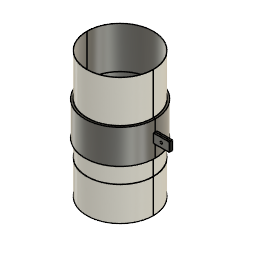
The Avionic Bay (Autodesk Fusion 360 design; units mm, degrees)
part number: 2026-03-09-17-46-28-485
Autodesk Fusion 360 part; units mm, degrees
sketch "Sketch1" plane through (0, 0, 0) normal (0, 0, 1) x (1, 0, 0)
  circle A0 centre (0, 0) radius 29.3705
  dimension "d1" = 58.741
  constraint coincident A0.centre origin
  measures "d1" diameter of A0
extrude "Extrude1" add sketch "Sketch1" along normal blind 112.014 makes body 1
shell "Shell1" thickness 0.1 removed faces 1 at (-8.7113, 2.7886, 112.014) on bodies 1
hole "Hole1" at (0, 0, 0) direction (0, 0, 1) diameter 58.74 depth 30 tip angle 118 bodies 1
sketch "Sketch2" plane through (0, 0, 0) normal (0, 1, 0) x (1, 0, 0)
split "Split1" by plane through (0, 0, 0) normal (0, 1, 0) bodies 1 makes body 2 at (-22.4991, 18.879, 37.338)
sketch "Sketch3" plane through (0, 0, 0) normal (0, 1, 0) x (1, 0, 0)
sketch "Sketch4" plane through (0, 0, 0) normal (0, 0, 1) x (1, 0, 0)
sketch "Sketch5" plane through (0, 0, 0) normal (0, 1, 0) x (1, 0, 0)
sketch "Sketch6" plane through (0, 0, 0) normal (0, 0, 1) x (1, 0, 0)
  circle A0 centre (0, 0) radius 31.0659
  constraint coincident A0.centre origin
extrude "Extrude2" add sketch "Sketch6" along normal blind 30 from surface at 45 separate body makes body 3
hole "Hole2" at (0, 0, 75) direction (0, 0, -1) diameter 58.74 depth 20 tip angle 118 bodies 1 2 3
delete_face "DeleteFace1" 1 faces at (-16.006, 20.0709, 52.7778) on bodies 3
split "Split2" by plane through (0, 0, 0) normal (0, 1, 0) bodies 3 makes body 4 at (-21.6913, 22.239, 65)
sketch "Sketch7" plane through (0, 0, 0) normal (0, 1, 0) x (1, 0, 0)
  line L0 (31, -65) -> (45, -65)
  line L1 (45, -65) -> (45, -57)
  line L2 (45, -57) -> (31, -57)
  line L3 (31, -57) -> (31, -65)
  circle A0 centre (38, -61) radius 1.016
  dimension "d14" = 2.032
  constraint horizontal L0
  constraint vertical L1
  constraint horizontal L2
  constraint vertical L3
  measures "d14" diameter of A0
extrude "Extrude3" add sketch "Sketch7" along normal blind 1.5 and the other way blind 1.5 separate body makes body 5
split "Split3" by plane through (0, 0, 0) normal (0, 1, 0) bodies 5 makes body 6 at (32.9947, 1.5, 61)
